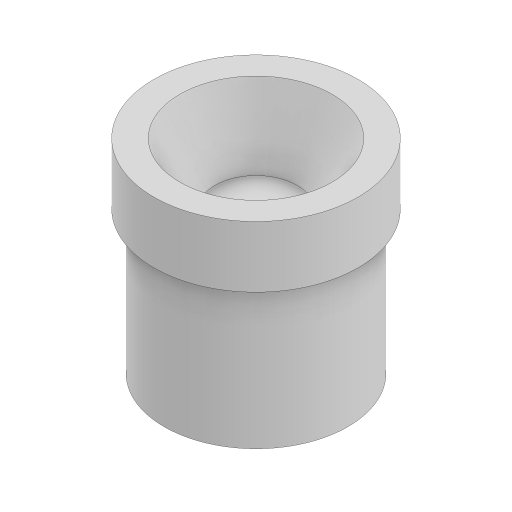
# Autodesk Inventor part: Magnethalter
Saved by Autodesk Inventor 2024.3 (Build 283343000, 343)
## iProperties
Created: 2025-05-15
Part Number: Magnethalter
Material: Generisch
Document SubType Name: Modeling
Designer: Demir
Density: 1 g/cm^3
Appearance: Vorgabe
Author: Demir
Autodesk Inventor part; units mm, degrees
ref_plane "YZ Plane" through (0, 0, 0) normal (1, 0, 0) x (0, 1, 0)
ref_plane "XZ Plane" through (0, 0, 0) normal (0, 1, 0) x (-1, 0, 0)
ref_plane "XY Plane" through (0, 0, 0) normal (0, 0, 1) x (1, 0, 0)
sketch "Skizze1" plane through (0, 0, 0) normal (0, 0, 1) x (1, 0, 0)
  circle A0 centre (0, 0) radius 22.5
  dimension "d0" = 45
  constraints: 1 centre point, 1 coincident
  measures "d0" diameter of A0
extrude "Extrusion1" add sketch "Skizze1" along normal mid plane 35
sketch "Skizze2" plane through (0, 0, 17.5) normal (0, 0, 1) x (1, 0, 0)
  circle A0 centre (0, 0) radius 22.5 projected
  circle A1 centre (0, 0) radius 25
  dimension "d3" = 50
  constraints: 1 centre point
  measures "d3" diameter of A1
extrude "Extrusion2" add sketch "Skizze2" along normal blind 15 contours A0 | A1
sketch "Skizze4" plane through (0, 0, 32.5) normal (0, 0, 1) x (1, 0, 0)
  circle A0 centre (0, 0) radius 25 projected
  circle A1 centre (0, 0) radius 10
  dimension "d6" = 20
  constraints: 1 centre point
  measures "d6" diameter of A1
extrude "Extrusion3" cut sketch "Skizze4" against normal blind 15 contours A1
chamfer "Fasen1" distance 15 angle 30 1 edges at (-10, 0, 32.5) measured on face at (9.9676, -0.8047, 22.5)
